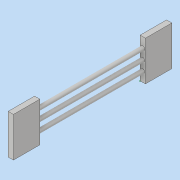
# Autodesk Inventor part: 2
Saved by Autodesk Inventor 2019 (Build 230136000, 136)
## iProperties
Created: 2020-02-15
Part Number: 2
Material: Generic
Document SubType Name: Modeling
Designer: Sudhanshu
Density: 1 g/cm^3
Appearance: Default
Author: Sudhanshu
Autodesk Inventor part; units mm, degrees
ref_plane "YZ Plane" through (0, 0, 0) normal (1, 0, 0) x (0, 1, 0)
ref_plane "XZ Plane" through (0, 0, 0) normal (0, 1, 0) x (-1, 0, 0)
ref_plane "XY Plane" through (0, 0, 0) normal (0, 0, 1) x (1, 0, 0)
sketch "Sketch1" plane through (0, 0, 0) normal (1, 0, 0) x (0, 1, 0)
  line L0 (0, 0) -> (0, -300)
  line L1 (0, -300) -> (0, 0)
  line L2 (0, 0) -> (0, 300)
  line L3 (0, 300) -> (150, 300)
  line L4 (150, 300) -> (150, 200)
  line L5 (150, 200) -> (0, 200)
  line L6 (0, 200) -> (0, 300)
  line L7 (0, -300) -> (150, -300)
  line L8 (150, -300) -> (150, -200)
  line L9 (150, -200) -> (0, -200)
  line L10 (0, -200) -> (0, -300)
  dimension "d0" = 300
  dimension "d1" = 300
  dimension "d2" = 150
  dimension "d3" = 100
  dimension "d4" = 150
  dimension "d5" = 100
  constraints: 22 end point, 5 equal length, 2 horizontal, 2 perpendicular, 2 vertical
  measures "d0" distance of L0.start L0.end
  measures "d1" distance of L0.start L2.end
  measures "d2" distance of L4.end L5.end
  measures "d3" distance of L3.end L4.end
  measures "d4" distance of L9.end L8.end
  measures "d5" distance of L8.end L7.end
extrude "Extrusion1" add sketch "Sketch1" along normal blind 20
sketch "Sketch2" plane through (0, 0, -200) normal (0, 0, 1) x (1, 0, 0)
  point P0 (0, 0)
sketch "Sketch6" plane through (0, 0, -200) normal (0, 0, 1) x (1, 0, 0)
  line L0 (0, 150) -> (20, 150) projected
  line L1 (10, 150) -> (10, 0)
  line L2 (10, 0) -> (10, 150)
  line L3 (10, 75) -> (10, 150)
  line L4 (10, 112.5) -> (10, 75)
  line L5 (10, 0) -> (10, 75)
  circle A0 centre (10, 112.5) radius 7.5
  circle A1 centre (10, 75) radius 7.5
  circle A2 centre (10, 37.5) radius 7.5
  point P0 (0, 0)
  dimension "d13" = 15
  dimension "d14" = 15
  dimension "d15" = 15
  constraints: 10 end point, 4 collinear, 4 midpoint, 3 centre point, 2 coincident, 1 vertical
  measures "d13" diameter of A0
  measures "d14" diameter of A1
  measures "d15" diameter of A2
extrude "Extrusion3" add sketch "Sketch6" along normal blind 400.125
body "Solid1"
